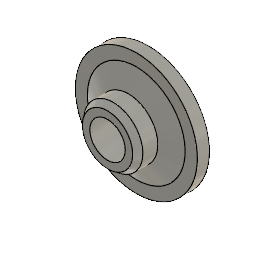
Hexapod (Autodesk Fusion 360 archive; units mm, degrees)
design "Servo Wheel"
Autodesk Fusion 360 part; units mm, degrees
sketch "Profile" plane through (-3.4, -2.5217, -2.4711) normal (-1, 0, 0) x (0, -1, 0)
  line L0 (-59, 21.875) -> (-59, 1.875)
  line L1 (-59, 1.875) -> (-57, 1.875)
  line L2 (-59, 21.875) -> (-57, 21.875)
  line L3 (-57, 21.875) -> (-57, 1.875)
  line L4 (-57, 19.875) -> (-57, 3.875)
  line L5 (-55.7, 16.7) -> (-55.7, 7.05)
  line L6 (-52.2841, 16) -> (-52.3159, 7.75)
  line L7 (-57, 11.875) -> (-55.7, 11.875) construction
  line L8 (-55.7, 11.875) -> (-52.3, 11.875) construction
  line L9 (-57, 19.875) -> (-55.7, 16.7)
  line L10 (-57, 3.875) -> (-55.7, 7.05)
  line L11 (-59, 11.875) -> (-52.3, 11.875)
  line L12 (-55.7, 16.7) -> (-53.2488, 16.7)
  line L13 (-53.2488, 16.7) -> (-52.2841, 16)
  line L14 (-55.7, 7.05) -> (-53.2715, 7.05)
  line L15 (-53.2715, 7.05) -> (-52.3159, 7.75)
  line L16 (-59, 11.875) -> (-52.3, 11.875) construction
  dimension "d77" = 20
  dimension "d78" = 2
  dimension "d79" = 16
  dimension "d80" = 9.65
  dimension "d81" = 8.25
  dimension "d82" = 2
  dimension "d83" = 1.3
  dimension "d84" = 3.4
  dimension "d86" = 0
  dimension "d87" = 0
  dimension "d88" = 0
  dimension "d89" = 0
  dimension "d107" = 0
  dimension "d108" = 0
  dimension "d109" = 0
  dimension "d110" = 0
  dimension "d126" = 0
  dimension "d127" = 0
  dimension "d128" = 0
  dimension "d129" = 0
  dimension "d149" = 0
  dimension "d150" = 0
  dimension "d151" = 0
  dimension "d152" = 0
  dimension "d1" = 6.4
  measures "d77" distance of origin
revolve "Revolve1" add sketch "Profile" angle 360 about axis through (-3.4, 56.4783, 9.4039) along (0, -1, 0) contours L0 L2 L3 L4 L11 | L3 L4 L5 L9 L11 | L5 L6 L11 L12 L13
sketch "Through Hole" plane through (0, 56.4783, 0) normal (0, 1, 0) x (-1, 0, 0)
  circle A0 centre (3.4, 9.4039) radius 10
  circle A1 centre (3.4, 9.4039) radius 2.9
  circle A2 centre (3.4, 9.4039) radius 1.25
  dimension "d98" = 5.8
  dimension "d103" = 2.5
  measures "d98" diameter of A1
  measures "d103" diameter of A2
extrude "Extrude1" cut sketch "Through Hole" against normal through all contours A2
extrude "Extrude2" cut sketch "Through Hole" against normal through all from surface at -2 contours A1

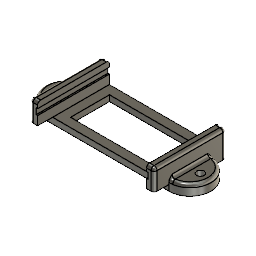
design "Receiver Holder"
Autodesk Fusion 360 part; units mm, degrees
sketch "Profile" plane through (0, 0, 0) normal (0, 1, 0) x (1, 0, 0)
  line L0 (11.5, 0) -> (11.5, -3)
  line L1 (11.5, -3) -> (12, -3)
  line L2 (12, -3) -> (12, -5)
  line L3 (12, -5) -> (11.5, -5)
  line L4 (11.5, -5) -> (11.5, -7)
  line L5 (11.5, -7) -> (14, -7)
  line L6 (14, -7) -> (14, 2)
  line L7 (14, 2) -> (-27.4, 2)
  line L8 (-27.4, 2) -> (-27.4, -7)
  line L9 (-27.4, -7) -> (-24.9, -7)
  line L10 (-24.9, -7) -> (-24.9, -5)
  line L11 (-24.9, -5) -> (-25.4, -5)
  line L12 (-25.4, -5) -> (-25.4, -3)
  line L13 (-25.4, -3) -> (-24.9, -3)
  line L14 (-24.9, -3) -> (-24.9, 0)
  line L15 (-24.9, 0) -> (11.5, 0)
  line L16 (-24.9, 0) -> (-27.4, 0)
  line L17 (11.5, 0) -> (14, 0)
  dimension "d3" = 3
  dimension "d4" = 0.5
  dimension "d5" = 2
  dimension "d6" = 0.5
  dimension "d7" = 2
  dimension "d8" = 2.5
  dimension "d9" = 9
  dimension "d10" = 41.4
  dimension "d11" = 9
  dimension "d12" = 2.5
  dimension "d13" = 2
  dimension "d14" = 0.5
  dimension "d15" = 2
  dimension "d16" = 0.5
  dimension "d33" = 3
extrude "Extrude1" add sketch "Profile" along normal blind 24
sketch "Bottom" plane through (0, 0, -2) normal (0, 0, -1) x (1, 0, 0)
  line L0 (14, 0) -> (-27.4, 0)
  line L1 (-27.4, 0) -> (-27.4, -24)
  line L2 (-27.4, -24) -> (14, -24)
  line L3 (14, -24) -> (14, 0)
  arc A0 (-27.4, -5) -> (-27.4, -19) centre (-27.4, -12) ccw
  arc A1 (14, -19) -> (14, -5) centre (14, -12) ccw
  line L4 (14, -12) -> (17.5, -12) construction
  line L5 (-27.4, -12) -> (-30.9, -12) construction
  circle A2 centre (-30.9, -12) radius 1.25
  circle A3 centre (17.5, -12) radius 1.25
  line L6 (-30.9, -12) -> (17.5, -12) construction
  line L7 (-6.7, -24) -> (-6.7, -21) construction
  line L8 (-27.4, -12) -> (-21.9, -12) construction
  line L9 (-6.7, 0) -> (-6.7, -8) construction
  line L10 (11.5, 0) -> (11.5, -24) construction
  line L11 (14, -12) -> (8.5, -12) construction
  line L12 (-21.9, -21) -> (8.5, -21)
  line L13 (8.5, -21) -> (8.5, -8)
  line L14 (8.5, -8) -> (-21.9, -8)
  line L15 (-21.9, -8) -> (-21.9, -21)
  line L16 (-21.9, -14.5) -> (8.5, -14.5) construction
  line L17 (-6.7, -14.5) -> (-6.7, -12) construction
  dimension "d19" = 7
  dimension "d20" = 7
  dimension "d21" = 3.5
  dimension "d22" = 3.5
  dimension "d23" = 2.5
  dimension "d24" = 2.5
  dimension "d29" = 35
  dimension "d38" = 3
  dimension "d39" = 5.5
  dimension "d40" = 8
  dimension "d41" = 5.5
  dimension "d42" = 13
  dimension "d43" = 30.4
  dimension "d45" = 2.5
  measures "d19" radius of A0
  measures "d20" radius of A1
  measures "d23" diameter of A2
  measures "d24" diameter of A3
  measures "d42" distance of origin
  measures "d43" distance of origin
extrude "Extrude2" add sketch "Bottom" against normal blind 3.5 contours L3 A1 | L1 A0
fillet "Fillet1" radius 1 4 edges at (-27.4, 12, 1.5) (-34.4, 12, 1.5) (14, 12, 1.5) (21, 12, 1.5)
fillet "Fillet2" radius 1 10 edges at (14, 12, 7) (14, 0, 2.5) (-27.4, 12, 7) (-27.4, 0, 2.5) (-26.15, 0, 7) (12.75, 0, 7) (12.75, 24, 7) (14, 24, 2.5) (-27.4, 24, 2.5) (-26.15, 24, 7)
extrude "Extrude3" cut sketch "Bottom" against normal blind 2 contours L12 L13 L14 L15
extrude "Extrude4" cut sketch "Profile" along normal blind 5 contours L6 L7 L8 L15 L16 L17
named bodies: "Receiver Holder"

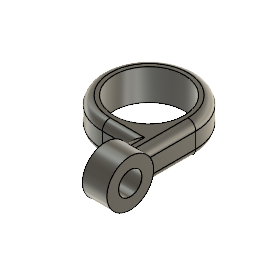
design "Wire Guide"
Autodesk Fusion 360 part; units mm, degrees
sketch "Profile" plane through (0, 0, 0) normal (0, 0, 1) x (1, 0, 0)
  line L0 (2.594, 0) -> (2.594, -6)
  line L1 (2.594, -6) -> (0, -6)
  line L2 (0, -6) -> (0, 0)
  circle A0 centre (-3.406, 6) radius 4.5
  line L3 (2.594, 6) -> (2.594, 0)
  line L4 (0, 0) -> (-3.406, 0)
  arc A1 (2.594, 6) -> (-3.406, 0) centre (-3.406, 6) ccw
  line L5 (2.594, -6) -> (3.175, -6)
  line L6 (3.175, -6) -> (3.175, 0)
  line L7 (3.175, 0) -> (2.594, 0)
  line L8 (2.594, 0) -> (2.594, -6)
  line L9 (3.175, -6) -> (0, -6) construction
  line L10 (0, -6) -> (0, 0) construction
  line L11 (0, 0) -> (3.175, 0) construction
  line L12 (3.175, 0) -> (3.175, -6) construction
  line L13 (2.594, -6) -> (-3.406, -6) construction
  line L14 (-3.406, -6) -> (-3.406, 6) construction
  line L15 (-3.406, 6) -> (2.594, 6) construction
  line L16 (2.594, 6) -> (2.594, -6) construction
  dimension "d38" = 6
  dimension "d39" = 6
  dimension "d40" = 0.581
  dimension "d42" = 6
  dimension "d43" = 3.175
  dimension "d44" = 12
  dimension "d45" = 6
  measures "d38" distance of L2.end
extrude "Extrude1" add sketch "Profile" along normal mid plane 6
sketch "Bottom" plane through (0, 0, 0) normal (1, 0, 0) x (0, 1, 0)
  line L0 (-6, -3) -> (-6, 3) construction
  circle A0 centre (-3, 0) radius 1.5
  circle A1 centre (-3, 0) radius 3
  line L1 (0, -3) -> (12, -3)
  line L2 (12, -3) -> (12, -2)
  line L3 (12, -2) -> (0, -2)
  line L4 (0, -2) -> (0, -3)
  line L5 (0, 3) -> (12, 3)
  line L6 (12, 3) -> (12, 2)
  line L7 (12, 2) -> (0, 2)
  line L8 (0, 2) -> (0, 3)
  line L9 (0, 0) -> (-3, 0) construction
  dimension "d9" = 3
  dimension "d28" = 6
  dimension "d31" = 12
  dimension "d32" = 1
  dimension "d33" = 12
  dimension "d34" = 1
  dimension "d37" = 3
  measures "d9" diameter of A0
  measures "d28" diameter of A1
  measures "d37" distance of L9.start
extrude "Extrude2" cut sketch "Bottom" along normal through all contours A0
extrude "Extrude3" cut sketch "Bottom" along normal through all and the other way through all contours L1 L2 L3 L4 | L5 L6 L7 L8
fillet "Fillet6" radius 3 4 edges at (1.5875, -6, 3) (1.5875, 0, 3) (1.5875, -6, -3) (1.5875, 0, -3)
fillet "Fillet3" radius 1 8 edges at (2.594, 2.618, -2) (-7.6486, 10.2426, -2) (-1.703, 0, -2) (-1.703, 0, 2) (-7.6486, 10.2426, 2) (2.594, 2.618, 2) (0, -0.382, -2) (0, -0.382, 2)
named bodies: "Wire Guide"

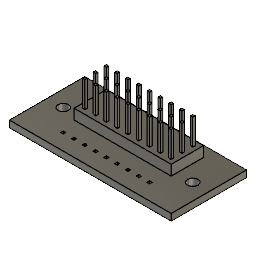
design "Servo Header"
Autodesk Fusion 360 part; units mm, degrees
sketch "Sketch1" plane through (0, 0, 0) normal (0, 0, 1) x (1, 0, 0)
  line L0 (0, 0) -> (2.54, 0)
  line L1 (2.54, 0) -> (2.54, 2.54)
  line L2 (2.54, 2.54) -> (0, 2.54)
  line L3 (0, 2.54) -> (0, 0)
  line L4 (1.57, 0.97) -> (0.97, 0.97)
  line L5 (0.97, 0.97) -> (0.97, 1.57)
  line L6 (0.97, 1.57) -> (1.57, 1.57)
  line L7 (1.57, 1.57) -> (1.57, 0.97)
  line L8 (1.57, 0.97) -> (0.97, 1.57) construction
  line L9 (0.97, 0.97) -> (1.57, 1.57) construction
  line L10 (3.51, 1.57) -> (4.11, 1.57)
  line L11 (3.51, 0.97) -> (4.11, 1.57) construction
  line L12 (4.11, 0.97) -> (3.51, 1.57) construction
  line L13 (4.11, 0.97) -> (3.51, 0.97)
  line L14 (5.08, 0) -> (5.08, 2.54)
  line L15 (3.51, 0.97) -> (3.51, 1.57)
  line L16 (5.08, 2.54) -> (2.54, 2.54)
  line L17 (2.54, 0) -> (5.08, 0)
  line L18 (2.54, 2.54) -> (2.54, 0)
  line L19 (4.11, 1.57) -> (4.11, 0.97)
  line L20 (6.05, 1.57) -> (6.65, 1.57)
  line L21 (6.05, 0.97) -> (6.65, 1.57) construction
  line L22 (6.65, 0.97) -> (6.05, 1.57) construction
  line L23 (6.65, 0.97) -> (6.05, 0.97)
  line L24 (7.62, 0) -> (7.62, 2.54)
  line L25 (6.05, 0.97) -> (6.05, 1.57)
  line L26 (7.62, 2.54) -> (5.08, 2.54)
  line L27 (5.08, 0) -> (7.62, 0)
  line L28 (5.08, 2.54) -> (5.08, 0)
  line L29 (6.65, 1.57) -> (6.65, 0.97)
  line L30 (8.59, 1.57) -> (9.19, 1.57)
  line L31 (8.59, 0.97) -> (9.19, 1.57) construction
  line L32 (9.19, 0.97) -> (8.59, 1.57) construction
  line L33 (9.19, 0.97) -> (8.59, 0.97)
  line L34 (10.16, 0) -> (10.16, 2.54)
  line L35 (8.59, 0.97) -> (8.59, 1.57)
  line L36 (10.16, 2.54) -> (7.62, 2.54)
  line L37 (7.62, 0) -> (10.16, 0)
  line L38 (7.62, 2.54) -> (7.62, 0)
  line L39 (9.19, 1.57) -> (9.19, 0.97)
  line L40 (11.13, 1.57) -> (11.73, 1.57)
  line L41 (11.13, 0.97) -> (11.73, 1.57) construction
  line L42 (11.73, 0.97) -> (11.13, 1.57) construction
  line L43 (11.73, 0.97) -> (11.13, 0.97)
  line L44 (12.7, 0) -> (12.7, 2.54)
  line L45 (11.13, 0.97) -> (11.13, 1.57)
  line L46 (12.7, 2.54) -> (10.16, 2.54)
  line L47 (10.16, 0) -> (12.7, 0)
  line L48 (10.16, 2.54) -> (10.16, 0)
  line L49 (11.73, 1.57) -> (11.73, 0.97)
  line L50 (13.67, 1.57) -> (14.27, 1.57)
  line L51 (13.67, 0.97) -> (14.27, 1.57) construction
  line L52 (14.27, 0.97) -> (13.67, 1.57) construction
  line L53 (14.27, 0.97) -> (13.67, 0.97)
  line L54 (15.24, 0) -> (15.24, 2.54)
  line L55 (13.67, 0.97) -> (13.67, 1.57)
  line L56 (15.24, 2.54) -> (12.7, 2.54)
  line L57 (12.7, 0) -> (15.24, 0)
  line L58 (12.7, 2.54) -> (12.7, 0)
  line L59 (14.27, 1.57) -> (14.27, 0.97)
  line L60 (16.21, 1.57) -> (16.81, 1.57)
  line L61 (16.21, 0.97) -> (16.81, 1.57) construction
  line L62 (16.81, 0.97) -> (16.21, 1.57) construction
  line L63 (16.81, 0.97) -> (16.21, 0.97)
  line L64 (17.78, 0) -> (17.78, 2.54)
  line L65 (16.21, 0.97) -> (16.21, 1.57)
  line L66 (17.78, 2.54) -> (15.24, 2.54)
  line L67 (15.24, 0) -> (17.78, 0)
  line L68 (15.24, 2.54) -> (15.24, 0)
  line L69 (16.81, 1.57) -> (16.81, 0.97)
  line L70 (18.75, 1.57) -> (19.35, 1.57)
  line L71 (18.75, 0.97) -> (19.35, 1.57) construction
  line L72 (19.35, 0.97) -> (18.75, 1.57) construction
  line L73 (19.35, 0.97) -> (18.75, 0.97)
  line L74 (20.32, 0) -> (20.32, 2.54)
  line L75 (18.75, 0.97) -> (18.75, 1.57)
  line L76 (20.32, 2.54) -> (17.78, 2.54)
  line L77 (17.78, 0) -> (20.32, 0)
  line L78 (17.78, 2.54) -> (17.78, 0)
  line L79 (19.35, 1.57) -> (19.35, 0.97)
  line L80 (21.29, 1.57) -> (21.89, 1.57)
  line L81 (21.29, 0.97) -> (21.89, 1.57) construction
  line L82 (21.89, 0.97) -> (21.29, 1.57) construction
  line L83 (21.89, 0.97) -> (21.29, 0.97)
  line L84 (22.86, 0) -> (22.86, 2.54)
  line L85 (21.29, 0.97) -> (21.29, 1.57)
  line L86 (22.86, 2.54) -> (20.32, 2.54)
  line L87 (20.32, 0) -> (22.86, 0)
  line L88 (20.32, 2.54) -> (20.32, 0)
  line L89 (21.89, 1.57) -> (21.89, 0.97)
  line L90 (0.97, 4.11) -> (1.57, 4.11)
  line L91 (0.97, 3.51) -> (1.57, 4.11) construction
  line L92 (1.57, 3.51) -> (0.97, 4.11) construction
  line L93 (1.57, 3.51) -> (0.97, 3.51)
  line L94 (2.54, 2.54) -> (2.54, 5.08)
  line L95 (0.97, 3.51) -> (0.97, 4.11)
  line L96 (2.54, 5.08) -> (0, 5.08)
  line L97 (0, 2.54) -> (2.54, 2.54)
  line L98 (0, 5.08) -> (0, 2.54)
  line L99 (1.57, 4.11) -> (1.57, 3.51)
  line L100 (3.51, 4.11) -> (4.11, 4.11)
  line L101 (3.51, 3.51) -> (4.11, 4.11) construction
  line L102 (4.11, 3.51) -> (3.51, 4.11) construction
  line L103 (4.11, 3.51) -> (3.51, 3.51)
  line L104 (5.08, 2.54) -> (5.08, 5.08)
  line L105 (3.51, 3.51) -> (3.51, 4.11)
  line L106 (5.08, 5.08) -> (2.54, 5.08)
  line L107 (2.54, 2.54) -> (5.08, 2.54)
  line L108 (2.54, 5.08) -> (2.54, 2.54)
  line L109 (4.11, 4.11) -> (4.11, 3.51)
  line L110 (6.05, 4.11) -> (6.65, 4.11)
  line L111 (6.05, 3.51) -> (6.65, 4.11) construction
  line L112 (6.65, 3.51) -> (6.05, 4.11) construction
  line L113 (6.65, 3.51) -> (6.05, 3.51)
  line L114 (7.62, 2.54) -> (7.62, 5.08)
  line L115 (6.05, 3.51) -> (6.05, 4.11)
  line L116 (7.62, 5.08) -> (5.08, 5.08)
  line L117 (5.08, 2.54) -> (7.62, 2.54)
  line L118 (5.08, 5.08) -> (5.08, 2.54)
  line L119 (6.65, 4.11) -> (6.65, 3.51)
  line L120 (8.59, 4.11) -> (9.19, 4.11)
  line L121 (8.59, 3.51) -> (9.19, 4.11) construction
  line L122 (9.19, 3.51) -> (8.59, 4.11) construction
  line L123 (9.19, 3.51) -> (8.59, 3.51)
  line L124 (10.16, 2.54) -> (10.16, 5.08)
  line L125 (8.59, 3.51) -> (8.59, 4.11)
  line L126 (10.16, 5.08) -> (7.62, 5.08)
  line L127 (7.62, 2.54) -> (10.16, 2.54)
  line L128 (7.62, 5.08) -> (7.62, 2.54)
  line L129 (9.19, 4.11) -> (9.19, 3.51)
  line L130 (11.13, 4.11) -> (11.73, 4.11)
  line L131 (11.13, 3.51) -> (11.73, 4.11) construction
  line L132 (11.73, 3.51) -> (11.13, 4.11) construction
  line L133 (11.73, 3.51) -> (11.13, 3.51)
  line L134 (12.7, 2.54) -> (12.7, 5.08)
  line L135 (11.13, 3.51) -> (11.13, 4.11)
  line L136 (12.7, 5.08) -> (10.16, 5.08)
  line L137 (10.16, 2.54) -> (12.7, 2.54)
  line L138 (10.16, 5.08) -> (10.16, 2.54)
  line L139 (11.73, 4.11) -> (11.73, 3.51)
  line L140 (13.67, 4.11) -> (14.27, 4.11)
  line L141 (13.67, 3.51) -> (14.27, 4.11) construction
  line L142 (14.27, 3.51) -> (13.67, 4.11) construction
  line L143 (14.27, 3.51) -> (13.67, 3.51)
  line L144 (15.24, 2.54) -> (15.24, 5.08)
  line L145 (13.67, 3.51) -> (13.67, 4.11)
  line L146 (15.24, 5.08) -> (12.7, 5.08)
  line L147 (12.7, 2.54) -> (15.24, 2.54)
  line L148 (12.7, 5.08) -> (12.7, 2.54)
  line L149 (14.27, 4.11) -> (14.27, 3.51)
  line L150 (16.21, 4.11) -> (16.81, 4.11)
  line L151 (16.21, 3.51) -> (16.81, 4.11) construction
  line L152 (16.81, 3.51) -> (16.21, 4.11) construction
  line L153 (16.81, 3.51) -> (16.21, 3.51)
  line L154 (17.78, 2.54) -> (17.78, 5.08)
  line L155 (16.21, 3.51) -> (16.21, 4.11)
  line L156 (17.78, 5.08) -> (15.24, 5.08)
  line L157 (15.24, 2.54) -> (17.78, 2.54)
  line L158 (15.24, 5.08) -> (15.24, 2.54)
  line L159 (16.81, 4.11) -> (16.81, 3.51)
  line L160 (18.75, 4.11) -> (19.35, 4.11)
  line L161 (18.75, 3.51) -> (19.35, 4.11) construction
  line L162 (19.35, 3.51) -> (18.75, 4.11) construction
  line L163 (19.35, 3.51) -> (18.75, 3.51)
  line L164 (20.32, 2.54) -> (20.32, 5.08)
  line L165 (18.75, 3.51) -> (18.75, 4.11)
  line L166 (20.32, 5.08) -> (17.78, 5.08)
  line L167 (17.78, 2.54) -> (20.32, 2.54)
  line L168 (17.78, 5.08) -> (17.78, 2.54)
  line L169 (19.35, 4.11) -> (19.35, 3.51)
  line L170 (21.29, 4.11) -> (21.89, 4.11)
  line L171 (21.29, 3.51) -> (21.89, 4.11) construction
  line L172 (21.89, 3.51) -> (21.29, 4.11) construction
  line L173 (21.89, 3.51) -> (21.29, 3.51)
  line L174 (22.86, 2.54) -> (22.86, 5.08)
  line L175 (21.29, 3.51) -> (21.29, 4.11)
  line L176 (22.86, 5.08) -> (20.32, 5.08)
  line L177 (20.32, 2.54) -> (22.86, 2.54)
  line L178 (20.32, 5.08) -> (20.32, 2.54)
  line L179 (21.89, 4.11) -> (21.89, 3.51)
  line L180 (0.97, 6.65) -> (1.57, 6.65)
  line L181 (0.97, 6.05) -> (1.57, 6.65) construction
  line L182 (1.57, 6.05) -> (0.97, 6.65) construction
  line L183 (1.57, 6.05) -> (0.97, 6.05)
  line L184 (2.54, 5.08) -> (2.54, 7.62)
  line L185 (0.97, 6.05) -> (0.97, 6.65)
  line L186 (2.54, 7.62) -> (0, 7.62)
  line L187 (0, 5.08) -> (2.54, 5.08)
  line L188 (0, 7.62) -> (0, 5.08)
  line L189 (1.57, 6.65) -> (1.57, 6.05)
  line L190 (3.51, 6.65) -> (4.11, 6.65)
  line L191 (3.51, 6.05) -> (4.11, 6.65) construction
  line L192 (4.11, 6.05) -> (3.51, 6.65) construction
  line L193 (4.11, 6.05) -> (3.51, 6.05)
  line L194 (5.08, 5.08) -> (5.08, 7.62)
  line L195 (3.51, 6.05) -> (3.51, 6.65)
  line L196 (5.08, 7.62) -> (2.54, 7.62)
  line L197 (2.54, 5.08) -> (5.08, 5.08)
  line L198 (2.54, 7.62) -> (2.54, 5.08)
  line L199 (4.11, 6.65) -> (4.11, 6.05)
  line L200 (6.05, 6.65) -> (6.65, 6.65)
  line L201 (6.05, 6.05) -> (6.65, 6.65) construction
  line L202 (6.65, 6.05) -> (6.05, 6.65) construction
  line L203 (6.65, 6.05) -> (6.05, 6.05)
  line L204 (7.62, 5.08) -> (7.62, 7.62)
  line L205 (6.05, 6.05) -> (6.05, 6.65)
  line L206 (7.62, 7.62) -> (5.08, 7.62)
  line L207 (5.08, 5.08) -> (7.62, 5.08)
  line L208 (5.08, 7.62) -> (5.08, 5.08)
  line L209 (6.65, 6.65) -> (6.65, 6.05)
  line L210 (8.59, 6.65) -> (9.19, 6.65)
  line L211 (8.59, 6.05) -> (9.19, 6.65) construction
  line L212 (9.19, 6.05) -> (8.59, 6.65) construction
  line L213 (9.19, 6.05) -> (8.59, 6.05)
  line L214 (10.16, 5.08) -> (10.16, 7.62)
  line L215 (8.59, 6.05) -> (8.59, 6.65)
  line L216 (10.16, 7.62) -> (7.62, 7.62)
  line L217 (7.62, 5.08) -> (10.16, 5.08)
  line L218 (7.62, 7.62) -> (7.62, 5.08)
  line L219 (9.19, 6.65) -> (9.19, 6.05)
  line L220 (11.13, 6.65) -> (11.73, 6.65)
  line L221 (11.13, 6.05) -> (11.73, 6.65) construction
  line L222 (11.73, 6.05) -> (11.13, 6.65) construction
  line L223 (11.73, 6.05) -> (11.13, 6.05)
  line L224 (12.7, 5.08) -> (12.7, 7.62)
  line L225 (11.13, 6.05) -> (11.13, 6.65)
  line L226 (12.7, 7.62) -> (10.16, 7.62)
  line L227 (10.16, 5.08) -> (12.7, 5.08)
  line L228 (10.16, 7.62) -> (10.16, 5.08)
  line L229 (11.73, 6.65) -> (11.73, 6.05)
  line L230 (13.67, 6.65) -> (14.27, 6.65)
  line L231 (13.67, 6.05) -> (14.27, 6.65) construction
  line L232 (14.27, 6.05) -> (13.67, 6.65) construction
  line L233 (14.27, 6.05) -> (13.67, 6.05)
  line L234 (15.24, 5.08) -> (15.24, 7.62)
  line L235 (13.67, 6.05) -> (13.67, 6.65)
  line L236 (15.24, 7.62) -> (12.7, 7.62)
  line L237 (12.7, 5.08) -> (15.24, 5.08)
  line L238 (12.7, 7.62) -> (12.7, 5.08)
  line L239 (14.27, 6.65) -> (14.27, 6.05)
  line L240 (16.21, 6.65) -> (16.81, 6.65)
  line L241 (16.21, 6.05) -> (16.81, 6.65) construction
  line L242 (16.81, 6.05) -> (16.21, 6.65) construction
  line L243 (16.81, 6.05) -> (16.21, 6.05)
  line L244 (17.78, 5.08) -> (17.78, 7.62)
  line L245 (16.21, 6.05) -> (16.21, 6.65)
  line L246 (17.78, 7.62) -> (15.24, 7.62)
  line L247 (15.24, 5.08) -> (17.78, 5.08)
  line L248 (15.24, 7.62) -> (15.24, 5.08)
  line L249 (16.81, 6.65) -> (16.81, 6.05)
  line L250 (18.75, 6.65) -> (19.35, 6.65)
  line L251 (18.75, 6.05) -> (19.35, 6.65) construction
  line L252 (19.35, 6.05) -> (18.75, 6.65) construction
  line L253 (19.35, 6.05) -> (18.75, 6.05)
  line L254 (20.32, 5.08) -> (20.32, 7.62)
  line L255 (18.75, 6.05) -> (18.75, 6.65)
  line L256 (20.32, 7.62) -> (17.78, 7.62)
  line L257 (17.78, 5.08) -> (20.32, 5.08)
  line L258 (17.78, 7.62) -> (17.78, 5.08)
  line L259 (19.35, 6.65) -> (19.35, 6.05)
  line L260 (21.29, 6.65) -> (21.89, 6.65)
  line L261 (21.29, 6.05) -> (21.89, 6.65) construction
  line L262 (21.89, 6.05) -> (21.29, 6.65) construction
  line L263 (21.89, 6.05) -> (21.29, 6.05)
  line L264 (22.86, 5.08) -> (22.86, 7.62)
  line L265 (21.29, 6.05) -> (21.29, 6.65)
  line L266 (22.86, 7.62) -> (20.32, 7.62)
  line L267 (20.32, 5.08) -> (22.86, 5.08)
  line L268 (20.32, 7.62) -> (20.32, 5.08)
  line L269 (21.89, 6.65) -> (21.89, 6.05)
  line L270 (0, 0) -> (0, -7.62) construction
  line L271 (0, 7.62) -> (0, 10.16) construction
  line L272 (22.86, 0) -> (30.48, 0) construction
  line L273 (0, 0) -> (-7.62, 0) construction
  line L274 (-7.62, -7.62) -> (30.48, -7.62)
  line L275 (30.48, -7.62) -> (30.48, 10.16)
  line L276 (30.48, 10.16) -> (-7.62, 10.16)
  line L277 (-7.62, 10.16) -> (-7.62, -7.62)
  circle A0 centre (26.67, 1.27) radius 1.2
  circle A1 centre (-3.81, 1.27) radius 1.2
  line L278 (-7.62, 1.27) -> (-3.81, 1.27) construction
  line L279 (30.48, 1.27) -> (26.67, 1.27) construction
  line L280 (1.57, -4.11) -> (0.97, -3.51) construction
  line L281 (1.57, -3.51) -> (1.57, -4.11)
  line L282 (1.57, -4.11) -> (0.97, -4.11)
  line L283 (0.97, -4.11) -> (1.57, -3.51) construction
  line L284 (0.97, -4.11) -> (0.97, -3.51)
  line L285 (0.97, -3.51) -> (1.57, -3.51)
  line L286 (4.11, -4.11) -> (3.51, -4.11)
  line L287 (3.51, -3.51) -> (4.11, -3.51)
  line L288 (4.11, -4.11) -> (3.51, -3.51) construction
  line L289 (3.51, -4.11) -> (3.51, -3.51)
  line L290 (3.51, -4.11) -> (4.11, -3.51) construction
  line L291 (4.11, -3.51) -> (4.11, -4.11)
  line L292 (6.05, -3.51) -> (6.65, -3.51)
  line L293 (6.05, -4.11) -> (6.05, -3.51)
  line L294 (6.65, -4.11) -> (6.05, -3.51) construction
  line L295 (6.65, -3.51) -> (6.65, -4.11)
  line L296 (6.65, -4.11) -> (6.05, -4.11)
  line L297 (6.05, -4.11) -> (6.65, -3.51) construction
  line L298 (8.59, -4.11) -> (8.59, -3.51)
  line L299 (9.19, -3.51) -> (9.19, -4.11)
  line L300 (9.19, -4.11) -> (8.59, -3.51) construction
  line L301 (8.59, -4.11) -> (9.19, -3.51) construction
  line L302 (8.59, -3.51) -> (9.19, -3.51)
  line L303 (9.19, -4.11) -> (8.59, -4.11)
  line L304 (11.13, -4.11) -> (11.73, -3.51) construction
  line L305 (11.73, -3.51) -> (11.73, -4.11)
  line L306 (11.73, -4.11) -> (11.13, -3.51) construction
  line L307 (11.73, -4.11) -> (11.13, -4.11)
  line L308 (11.13, -4.11) -> (11.13, -3.51)
  line L309 (11.13, -3.51) -> (11.73, -3.51)
  line L310 (14.27, -4.11) -> (13.67, -4.11)
  line L311 (13.67, -4.11) -> (14.27, -3.51) construction
  line L312 (14.27, -4.11) -> (13.67, -3.51) construction
  line L313 (13.67, -3.51) -> (14.27, -3.51)
  line L314 (13.67, -4.11) -> (13.67, -3.51)
  line L315 (14.27, -3.51) -> (14.27, -4.11)
  line L316 (16.21, -4.11) -> (16.21, -3.51)
  line L317 (16.81, -3.51) -> (16.81, -4.11)
  line L318 (16.21, -4.11) -> (16.81, -3.51) construction
  line L319 (16.81, -4.11) -> (16.21, -4.11)
  line L320 (16.21, -3.51) -> (16.81, -3.51)
  line L321 (16.81, -4.11) -> (16.21, -3.51) construction
  line L322 (18.75, -4.11) -> (19.35, -3.51) construction
  line L323 (18.75, -3.51) -> (19.35, -3.51)
  line L324 (19.35, -3.51) -> (19.35, -4.11)
  line L325 (19.35, -4.11) -> (18.75, -3.51) construction
  line L326 (18.75, -4.11) -> (18.75, -3.51)
  line L327 (19.35, -4.11) -> (18.75, -4.11)
  line L328 (21.89, -4.11) -> (21.29, -4.11)
  line L329 (21.29, -4.11) -> (21.29, -3.51)
  line L330 (21.89, -3.51) -> (21.89, -4.11)
  line L331 (21.29, -3.51) -> (21.89, -3.51)
  line L332 (21.89, -4.11) -> (21.29, -3.51) construction
  line L333 (21.29, -4.11) -> (21.89, -3.51) construction
  point P0 (-350.72, -350.72)
  point P1 (0, -350.72)
  dimension "d9" = 7.62
  dimension "d10" = 2.54
  dimension "d12" = 7.62
  dimension "d13" = 7.62
  dimension "d16" = 2.4
  dimension "d17" = 2.4
  dimension "d24" = 3.81
  dimension "d25" = 3.81
  dimension "d28" = 0
  dimension "d29" = -5.08
  measures "d9" distance of L0.start
  measures "d13" distance of L0.start
  measures "d16" diameter of A0
  measures "d17" diameter of A1
extrude "Extrude1" add sketch "Sketch1" along normal blind 1.6 contours L274 L275 L276 L277 | L281 L282 L284 L285 | L286 L287 L289 L291 | L292 L293 L295 L296 | L298 L299 L302 L303 | L305 L307 L308 L309 | L310 L313 L314 L315 | L316 L317 L319 L320 | L323 L324 L326 L327 | L328 L329 L330 L331
extrude "Extrude2" add sketch "Sketch1" along normal blind 4 contours L0 L1 L2 L3 L18 L97 | L1 L14 L16 L17 L18 L28 L107 | L2 L94 L96 L97 L98 L108 L187 | L16 L94 L104 L106 L107 L108 L118 L197 | L14 L24 L26 L27 L28 L38 L117 | L96 L184 L186 L187 L188 L198 | L26 L104 L114 L116 L117 L118 L128 L207 | L106 L184 L194 L196 L197 L198 L208 | L24 L34 L36 L37 L38 L48 L127 | L36 L114 L124 L126 L127 L128 L138 L217 | L116 L194 L204 L206 L207 L208 L218 | L34 L44 L46 L47 L48 L58 L137 | L46 L124 L134 L136 L137 L138 L148 L227 | L126 L204 L214 L216 L217 L218 L228 | L44 L54 L56 L57 L58 L68 L147 | L56 L134 L144 L146 L147 L148 L158 L237 | L136 L214 L224 L226 L227 L228 L238 | L54 L64 L66 L67 L68 L78 L157 | L66 L144 L154 L156 L157 L158 L168 L247 | L146 L224 L234 L236 L237 L238 L248 | L64 L74 L76 L77 L78 L88 L167 | L76 L154 L164 L166 L167 L168 L178 L257 | L156 L234 L244 L246 L247 L248 L258 | L74 L84 L86 L87 L88 L177 | L86 L164 L174 L176 L177 L178 L267 | L166 L244 L254 L256 L257 L258 L268 | L176 L254 L264 L266 L267 L268
extrude "Extrude3" add sketch "Sketch1" along normal blind 10.1 contours L4 L5 L6 L7 | L10 L13 L15 L19 | L20 L23 L25 L29 | L30 L33 L35 L39 | L40 L43 L45 L49 | L50 L53 L55 L59 | L60 L63 L65 L69 | L70 L73 L75 L79 | L80 L83 L85 L89 | L90 L93 L95 L99 | L100 L103 L105 L109 | L110 L113 L115 L119 | L120 L123 L125 L129 | L130 L133 L135 L139 | L140 L143 L145 L149 | L150 L153 L155 L159 | L160 L163 L165 L169 | L170 L173 L175 L179 | L180 L183 L185 L189 | L190 L193 L195 L199 | L200 L203 L205 L209 | L210 L213 L215 L219 | L220 L223 L225 L229 | L230 L233 L235 L239 | L240 L243 L245 L249 | L250 L253 L255 L259 | L260 L263 L265 L269
extrude "Extrude4" cut sketch "Sketch1" along normal through all contours L281 L282 L284 L285 | L286 L287 L289 L291 | L292 L293 L295 L296 | L298 L299 L302 L303 | L305 L307 L308 L309 | L310 L313 L314 L315 | L316 L317 L319 L320 | L323 L324 L326 L327 | L328 L329 L330 L331
equation "d9 = 2.54 mm * 3"
equation "d12 = ( 2.54 * 3 ) * 1 mm"
equation "d13 = ( 2.54 * 3 ) * 1 mm"
equation "d20 = 1.6 mm + 2.4 mm"
equation "d22 = 1.6 mm + 8.5 mm"
equation "d24 = ( 2.54 * 1.5 ) * 1 mm"
equation "d25 = ( 2.54 * 1.5 ) * 1 mm"
equation "d29 = ( -2.54 * 2 ) * 1 mm"

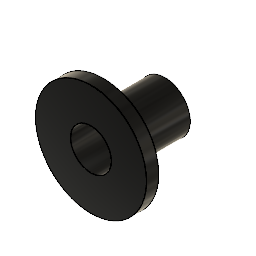
design "Bearing Center"
Autodesk Fusion 360 part; units mm, degrees
sketch "Sketch1" plane through (0, 0, 0) normal (0, 1, 0) x (1, 0, 0)
  circle A0 centre (0, 0) radius 2.05
  circle A1 centre (0, 0) radius 1.65
  circle A2 centre (0, 0) radius 4.5
  dimension "d1" = 4.1
  dimension "d2" = 3.3
  dimension "d3" = 9
  measures "d1" diameter of A0
  measures "d2" diameter of A1
  measures "d3" diameter of A2
extrude "Extrude1" add sketch "Sketch1" along normal blind 6 contours A0
extrude "Extrude2" add sketch "Sketch1" along normal blind 1 contours A2
named bodies: "Bearing Center"

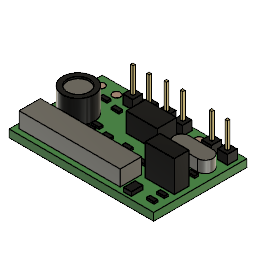
design "Receiver"
Autodesk Fusion 360 part; units mm, degrees
sketch "Sketch1" plane through (0, 0, 0) normal (0, 0, 1) x (1, 0, 0)
  line L0 (18.6, -12) -> (-18.6, -12)
  line L1 (-18.6, -12) -> (-18.6, 12)
  line L2 (-18.6, 12) -> (18.6, 12)
  line L3 (18.6, 12) -> (18.6, -12)
  line L4 (-18.6, -12) -> (-17.3635, -12) construction
  line L5 (-18.6, -10.65) -> (-18.6, -12) construction
  line L6 (-17.3635, -10.65) -> (8.6365, -10.65)
  line L7 (8.6365, -10.65) -> (8.6365, -5.15)
  line L8 (8.6365, -5.15) -> (-17.3635, -5.15)
  line L9 (-17.3635, -5.15) -> (-17.3635, -10.65)
  circle A0 centre (-13.3452, 0.5737) radius 4.075
  circle A1 centre (-13.3452, 0.5737) radius 2.8242
  line L10 (9.7824, -1.5868) -> (17.2824, -1.5868)
  line L11 (17.2824, -1.5868) -> (17.2824, -5.3868)
  line L12 (17.2824, -5.3868) -> (9.7824, -5.3868)
  line L13 (9.7824, -5.3868) -> (9.7824, -1.5868)
  line L14 (10.1467, -8.3154) -> (12.1467, -8.3154)
  line L15 (12.1467, -8.3154) -> (12.1467, -11.3154)
  line L16 (12.1467, -11.3154) -> (10.1467, -11.3154)
  line L17 (10.1467, -11.3154) -> (10.1467, -8.3154)
  line L18 (-7.0489, -3.1736) -> (-2.0489, -3.1736)
  line L19 (-2.0489, -3.1736) -> (-2.0489, -5.1736)
  line L20 (-2.0489, -5.1736) -> (-7.0489, -5.1736)
  line L21 (-7.0489, -5.1736) -> (-7.0489, -3.1736)
  line L22 (9.1707, 6.6458) -> (15.17, 6.6458)
  line L23 (17.17, 4.6511) -> (17.17, 4.6511)
  line L24 (15.17, 2.6458) -> (9.1707, 2.6458)
  line L25 (7.1707, 4.6401) -> (7.1707, 4.6401)
  arc A2 (9.1707, 6.6458) -> (7.1707, 4.6401) centre (9.1707, 4.6458) ccw
  arc A3 (7.1707, 4.6401) -> (9.1707, 2.6458) centre (9.1707, 4.6458) ccw
  arc A4 (17.17, 4.6511) -> (15.17, 6.6458) centre (15.17, 4.6458) ccw
  arc A5 (15.17, 2.6458) -> (17.17, 4.6511) centre (15.17, 4.6458) ccw
  line L26 (15.029, 7.9882) -> (17.569, 7.9882)
  line L27 (17.569, 7.9882) -> (17.569, 10.5282)
  line L28 (17.569, 10.5282) -> (15.029, 10.5282)
  line L29 (15.029, 10.5282) -> (15.029, 7.9882)
  line L30 (-5.2876, 10.5822) -> (-2.7476, 10.5822)
  line L31 (-2.7476, 10.5822) -> (-2.7476, 8.0422)
  line L32 (-2.7476, 8.0422) -> (-5.2876, 8.0422)
  line L33 (-5.2876, 8.0422) -> (-5.2876, 10.5822)
  line L34 (-9.3461, 10.5822) -> (-6.8061, 10.5822)
  line L35 (-6.8061, 10.5822) -> (-6.8061, 8.0422)
  line L36 (-6.8061, 8.0422) -> (-9.3461, 8.0422)
  line L37 (-9.3461, 8.0422) -> (-9.3461, 10.5822)
  line L38 (2.7807, 11.1689) -> (5.3207, 11.1689)
  line L39 (5.3207, 11.1689) -> (5.3207, 8.6289)
  line L40 (5.3207, 8.6289) -> (2.7807, 8.6289)
  line L41 (2.7807, 8.6289) -> (2.7807, 11.1689)
  line L42 (-1.3638, 11.2107) -> (1.1762, 11.2107)
  line L43 (1.1762, 11.2107) -> (1.1762, 8.6707)
  line L44 (1.1762, 8.6707) -> (-1.3638, 8.6707)
  line L45 (-1.3638, 8.6707) -> (-1.3638, 11.2107)
  line L46 (10.9956, 10.4785) -> (13.5356, 10.4785)
  line L47 (13.5356, 10.4785) -> (13.5356, 7.9385)
  line L48 (13.5356, 7.9385) -> (10.9956, 7.9385)
  line L49 (10.9956, 7.9385) -> (10.9956, 10.4785)
  line L50 (-2.5723, 7.0984) -> (5.4277, 7.0984)
  line L51 (5.4277, 7.0984) -> (5.4277, 2.0984)
  line L52 (5.4277, 2.0984) -> (-2.5723, 2.0984)
  line L53 (-2.5723, 2.0984) -> (-2.5723, 7.0984)
  circle A6 centre (-12.317, 9.3785) radius 1
  circle A7 centre (-16.3775, 9.3902) radius 1
  circle A8 centre (8.3691, 9.8873) radius 1
  line L54 (-13.7071, 7.3102) -> (-11.7071, 7.3102)
  line L55 (-11.7071, 7.3102) -> (-11.7071, 6.3102)
  line L56 (-11.7071, 6.3102) -> (-13.7071, 6.3102)
  line L57 (-13.7071, 6.3102) -> (-13.7071, 7.3102)
  line L58 (-9.7657, 6.4316) -> (-7.7657, 6.4316)
  line L59 (-7.7657, 6.4316) -> (-7.7657, 5.4316)
  line L60 (-7.7657, 5.4316) -> (-9.7657, 5.4316)
  line L61 (-9.7657, 5.4316) -> (-9.7657, 6.4316)
  line L62 (-8.8702, 0.4569) -> (-6.8702, 0.4569)
  line L63 (-6.8702, 0.4569) -> (-6.8702, -0.5431)
  line L64 (-6.8702, -0.5431) -> (-8.8702, -0.5431)
  line L65 (-8.8702, -0.5431) -> (-8.8702, 0.4569)
  line L66 (-9.1462, -1.1246) -> (-7.1462, -1.1246)
  line L67 (-7.1462, -1.1246) -> (-7.1462, -2.1246)
  line L68 (-7.1462, -2.1246) -> (-9.1462, -2.1246)
  line L69 (-9.1462, -2.1246) -> (-9.1462, -1.1246)
  line L70 (-10.0397, -2.7377) -> (-8.0397, -2.7377)
  line L71 (-8.0397, -2.7377) -> (-8.0397, -3.7377)
  line L72 (-8.0397, -3.7377) -> (-10.0397, -3.7377)
  line L73 (-10.0397, -3.7377) -> (-10.0397, -2.7377)
  line L74 (-5.0122, -0.656) -> (-3.0122, -0.656)
  line L75 (-3.0122, -0.656) -> (-3.0122, -1.656)
  line L76 (-3.0122, -1.656) -> (-5.0122, -1.656)
  line L77 (-5.0122, -1.656) -> (-5.0122, -0.656)
  line L78 (0.0422, -3.3505) -> (2.0422, -3.3505)
  line L79 (2.0422, -3.3505) -> (2.0422, -4.3505)
  line L80 (2.0422, -4.3505) -> (0.0422, -4.3505)
  line L81 (0.0422, -4.3505) -> (0.0422, -3.3505)
  line L82 (-0.0539, -0.5974) -> (1.9461, -0.5974)
  line L83 (1.9461, -0.5974) -> (1.9461, -1.5974)
  line L84 (1.9461, -1.5974) -> (-0.0539, -1.5974)
  line L85 (-0.0539, -1.5974) -> (-0.0539, -0.5974)
  line L86 (5.1762, -4.1119) -> (7.1762, -4.1119)
  line L87 (7.1762, -4.1119) -> (7.1762, -5.1119)
  line L88 (7.1762, -5.1119) -> (5.1762, -5.1119)
  line L89 (5.1762, -5.1119) -> (5.1762, -4.1119)
  line L90 (5.0934, -1.917) -> (7.0934, -1.917)
  line L91 (7.0934, -1.917) -> (7.0934, -2.917)
  line L92 (7.0934, -2.917) -> (5.0934, -2.917)
  line L93 (5.0934, -2.917) -> (5.0934, -1.917)
  line L94 (8.3737, 7.9822) -> (10.3737, 7.9822)
  line L95 (10.3737, 7.9822) -> (10.3737, 6.9822)
  line L96 (10.3737, 6.9822) -> (8.3737, 6.9822)
  line L97 (8.3737, 6.9822) -> (8.3737, 7.9822)
  line L98 (14.8169, -9.126) -> (16.8169, -9.126)
  line L99 (16.8169, -9.126) -> (16.8169, -10.126)
  line L100 (16.8169, -10.126) -> (14.8169, -10.126)
  line L101 (14.8169, -10.126) -> (14.8169, -9.126)
  line L102 (14.8755, -6.5445) -> (16.8755, -6.5445)
  line L103 (16.8755, -6.5445) -> (16.8755, -7.5445)
  line L104 (16.8755, -7.5445) -> (14.8755, -7.5445)
  line L105 (14.8755, -7.5445) -> (14.8755, -6.5445)
  line L106 (14.2898, 1.8318) -> (16.2898, 1.8318)
  line L107 (16.2898, 1.8318) -> (16.2898, 0.8318)
  line L108 (16.2898, 0.8318) -> (14.2898, 0.8318)
  line L109 (14.2898, 0.8318) -> (14.2898, 1.8318)
  line L110 (5.7378, 2.2418) -> (6.7378, 2.2418)
  line L111 (6.7378, 2.2418) -> (6.7378, 0.2418)
  line L112 (6.7378, 0.2418) -> (5.7378, 0.2418)
  line L113 (5.7378, 0.2418) -> (5.7378, 2.2418)
  line L114 (5.8549, 5.3463) -> (6.8549, 5.3463)
  line L115 (6.8549, 5.3463) -> (6.8549, 3.3463)
  line L116 (6.8549, 3.3463) -> (5.8549, 3.3463)
  line L117 (5.8549, 3.3463) -> (5.8549, 5.3463)
  line L118 (5.9135, 7.8651) -> (6.9135, 7.8651)
  line L119 (6.9135, 7.8651) -> (6.9135, 5.8651)
  line L120 (6.9135, 5.8651) -> (5.9135, 5.8651)
  line L121 (5.9135, 5.8651) -> (5.9135, 7.8651)
  line L122 (-17.3635, -3.4986) -> (-15.3635, -3.4986)
  line L123 (-15.3635, -3.4986) -> (-15.3635, -4.4986)
  line L124 (-15.3635, -4.4986) -> (-17.3635, -4.4986)
  line L125 (-17.3635, -4.4986) -> (-17.3635, -3.4986)
  line L126 (-8.353, 9.6467) -> (-7.703, 9.6467)
  line L127 (-7.703, 9.6467) -> (-7.703, 8.9967)
  line L128 (-7.703, 8.9967) -> (-8.353, 8.9967)
  line L129 (-8.353, 8.9967) -> (-8.353, 9.6467)
  line L130 (-3.6201, 9.0505) -> (-4.2701, 9.0505)
  line L131 (-4.2701, 9.0505) -> (-4.2701, 9.7005)
  line L132 (-3.6201, 9.7005) -> (-3.6201, 9.0505)
  line L133 (-4.2701, 9.7005) -> (-3.6201, 9.7005)
  line L134 (0.2479, 9.6414) -> (-0.4021, 9.6414)
  line L135 (0.2479, 10.2914) -> (0.2479, 9.6414)
  line L136 (3.7882, 10.2914) -> (4.4382, 10.2914)
  line L137 (4.4382, 9.6414) -> (3.7882, 9.6414)
  line L138 (4.4382, 10.2914) -> (4.4382, 9.6414)
  line L139 (-0.4021, 9.6414) -> (-0.4021, 10.2914)
  line L140 (3.7882, 9.6414) -> (3.7882, 10.2914)
  line L141 (-0.4021, 10.2914) -> (0.2479, 10.2914)
  line L142 (11.9539, 9.593) -> (12.6039, 9.593)
  line L143 (12.6039, 8.943) -> (11.9539, 8.943)
  line L144 (16.0367, 8.8893) -> (16.0367, 9.5393)
  line L145 (11.9539, 8.943) -> (11.9539, 9.593)
  line L146 (16.6867, 8.8893) -> (16.0367, 8.8893)
  line L147 (16.0367, 9.5393) -> (16.6867, 9.5393)
  line L148 (16.6867, 9.5393) -> (16.6867, 8.8893)
  line L149 (12.6039, 9.593) -> (12.6039, 8.943)
extrude "Extrude1" add sketch "Sketch1" along normal blind 2 contours L0 L1 L2 L3 makes body 1
extrude "Extrude2" add sketch "Sketch1" along normal blind 2.5 separate body contours L54 L55 L56 L57 | L58 L59 L60 L61 | L62 L63 L64 L65 | L66 L67 L68 L69 | L70 L71 L72 L73 | L74 L75 L76 L77 | L78 L79 L80 L81 | L82 L83 L84 L85 | L86 L87 L88 L89 | L90 L91 L92 L93 | L94 L95 L96 L97 | L98 L99 L100 L101 | L102 L103 L104 L105 | L106 L107 L108 L109 | L110 L111 L112 L113 | L114 L115 L116 L117 | L118 L119 L120 L121 | L122 L123 L124 L125 makes body 2 at (-16.6968, -3.4986, 0.8333) makes body 3 at (-4.3455, -0.656, 0.8333) makes body 4 at (5.7601, -1.917, 0.8333) makes body 5 at (6.8549, 4.6797, 0.8333) makes body 6 at (-13.0405, 7.3102, 0.8333) makes body 7 at (6.7378, 1.5752, 0.8333) makes body 8 at (5.8429, -4.1119, 0.8333) makes body 9 at (-8.2035, 0.4569, 0.8333) makes body 10 at (15.5422, -6.5445, 0.8333) makes body 11 at (-9.373, -2.7377, 0.8333) makes body 12 at (0.6128, -0.5974, 0.8333) makes body 13 at (14.9564, 1.8318, 0.8333) makes body 14 at (6.9135, 7.1984, 0.8333) makes body 15 at (-9.099, 6.4316, 0.8333) makes body 16 at (9.0403, 7.9822, 0.8333) makes body 17 at (0.7089, -3.3505, 0.8333) makes body 18 at (-8.4795, -1.1246, 0.8333) makes body 19 at (15.4836, -9.126, 0.8333)
extrude "Extrude3" add sketch "Sketch1" along normal blind 11 separate body contours L126 L127 L128 L129 | L130 L131 L132 L133 | L134 L135 L139 L141 | L136 L137 L138 L140 | L142 L143 L145 L149 | L144 L146 L147 L148 makes body 20 at (4.4382, 10.0747, 3.6667) makes body 21 at (-8.353, 9.2134, 3.6667) makes body 22 at (12.1705, 9.593, 3.6667) makes body 23 at (0.2479, 10.0747, 3.6667) makes body 24 at (-3.6201, 9.4838, 3.6667) makes body 25 at (16.0367, 9.106, 3.6667)
extrude "Extrude4" add sketch "Sketch1" along normal blind 4.4 separate body contours L26 L27 L28 L29 | L30 L31 L32 L33 | L34 L35 L36 L37 | L38 L39 L40 L41 | L42 L43 L44 L45 | L46 L47 L48 L49 makes body 26 at (3.6273, 11.1689, 1.4667) makes body 27 at (-8.4995, 10.5822, 1.4667) makes body 28 at (13.5356, 9.6319, 1.4667) makes body 29 at (-0.5171, 11.2107, 1.4667) makes body 30 at (-4.4409, 10.5822, 1.4667) makes body 31 at (15.029, 9.6815, 1.4667)
extrude "Extrude5" add sketch "Sketch1" along normal blind 2.1 separate body contours A6 | A7 | A8 makes body 32 at (9.3641, 9.7877, 0.7) makes body 33 at (-11.322, 9.2789, 0.7) makes body 34 at (-15.3825, 9.2907, 0.7)
extrude "Extrude6" add sketch "Sketch1" along normal blind 8 separate body contours A0 makes body 35
extrude "Extrude7" add sketch "Sketch1" along normal blind 7.5 separate body contours A1 makes body 36
extrude "Extrude8" add sketch "Sketch1" along normal blind 7 separate body contours L50 L51 L52 L53 makes body 37
extrude "Extrude9" add sketch "Sketch1" along normal blind 5 separate body contours L22 L24 A2 A3 A4 A5 makes body 38
extrude "Extrude10" add sketch "Sketch1" along normal blind 10 separate body contours L10 L11 L12 L13 makes body 39
extrude "Extrude11" add sketch "Sketch1" along normal blind 6 separate body contours L6 L7 L8 L9 L19 L20 L21 makes body 40
extrude "Extrude12" add sketch "Sketch1" along normal blind 3 separate body contours L8 L18 L19 L21 | L14 L15 L16 L17 makes body 41 at (-5.3822, -3.1736, 1) makes body 42 at (12.1467, -9.3154, 1)

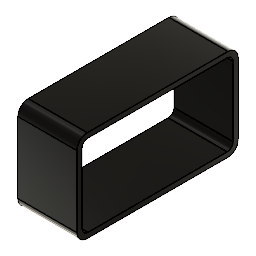
design "Battery Strap"
Autodesk Fusion 360 part; units mm, degrees
sketch "Sketch1" plane through (0, 0, 0) normal (1, 0, 0) x (0, 1, 0)
  line L0 (23.5, -13.75) -> (-23.5, -13.75)
  line L1 (-25.5, -11.75) -> (-25.5, 11.75)
  line L2 (-23.5, 13.75) -> (23.5, 13.75)
  line L3 (25.5, 11.75) -> (25.5, -11.75)
  line L4 (25.5, -13.75) -> (-25.5, 13.75) construction
  line L5 (-25.5, -13.75) -> (25.5, 13.75) construction
  line L6 (23.75, -15.5) -> (-23.75, -15.5)
  line L7 (-27.25, -12) -> (-27.25, 12)
  line L8 (-23.75, 15.5) -> (23.75, 15.5)
  line L9 (27.25, 12) -> (27.25, -12)
  line L10 (27.25, -15.5) -> (-27.25, 15.5) construction
  line L11 (-27.25, -15.5) -> (27.25, 15.5) construction
  arc A0 (27.25, 12) -> (23.75, 15.5) centre (23.75, 12) ccw
  arc A1 (23.75, -15.5) -> (27.25, -12) centre (23.75, -12) ccw
  arc A2 (-27.25, -12) -> (-23.75, -15.5) centre (-23.75, -12) ccw
  arc A3 (-23.75, 15.5) -> (-27.25, 12) centre (-23.75, 12) ccw
  arc A4 (-23.5, 13.75) -> (-25.5, 11.75) centre (-23.5, 11.75) ccw
  arc A5 (25.5, 11.75) -> (23.5, 13.75) centre (23.5, 11.75) ccw
  arc A6 (23.5, -13.75) -> (25.5, -11.75) centre (23.5, -11.75) ccw
  arc A7 (-25.5, -11.75) -> (-23.5, -13.75) centre (-23.5, -11.75) ccw
  dimension "d1" = 51
  dimension "d2" = 27.5
  dimension "d3" = 54.5
  dimension "d4" = 31
  dimension "d7" = 3.5
  dimension "d8" = 3.5
  dimension "d9" = 3.5
  dimension "d10" = 3.5
  dimension "d11" = 2
  dimension "d12" = 2
  dimension "d13" = 2
  dimension "d14" = 2
  measures "d7" radius of A0
  measures "d8" radius of A1
  measures "d9" radius of A2
  measures "d10" radius of A3
  measures "d11" radius of A4
  measures "d12" radius of A5
  measures "d13" radius of A6
  measures "d14" radius of A7
extrude "Extrude1" add sketch "Sketch1" along normal mid plane 20
equation "d3 = 51 mm + 1.75 mm + 1.75 mm"
equation "d4 = 27.5 mm + 1.75 mm + 1.75 mm"
named bodies: "Battery Strap"

design "624Z Bearing"
Autodesk Fusion 360 part; units mm, degrees
sketch "Sketch1" plane through (0.0608, -5, -3.3084) normal (0, -1, 0) x (1, 0, 0)
  circle A0 centre (9.4392, 13.5084) radius 6.5
  circle A1 centre (9.4392, 13.5084) radius 2
  circle A2 centre (9.4392, 13.5084) radius 3
  circle A3 centre (9.4392, 13.5084) radius 5.5
  circle A4 centre (9.4392, 13.5084) radius 5.2
  circle A5 centre (9.4392, 13.5084) radius 3.25
  dimension "d44" = 13
  dimension "d45" = 4
  dimension "d46" = 6
  dimension "d47" = 11
  dimension "d48" = 10.4
  dimension "d49" = 6.5
  dimension "d56" = 0
  dimension "d57" = 0
  dimension "d58" = 0
  dimension "d59" = 0
  dimension "d68" = 0
  dimension "d69" = 0
  dimension "d70" = 0
  dimension "d71" = 0
  measures "d44" diameter of A0
  measures "d45" diameter of A1
  measures "d46" diameter of A2
  measures "d47" diameter of A3
  measures "d48" diameter of A4
  measures "d49" diameter of A5
extrude "Extrude1" add sketch "Sketch1" along normal mid plane 5 contours A0 | A2 makes body 1 at (15.9919, -6.6667, 9.876) makes body 2 at (12.4963, -6.6667, 10.0505)
extrude "Extrude2" add sketch "Sketch1" along normal mid plane 4.8 separate body contours A4 makes body 3
extrude "Extrude3" add sketch "Sketch1" along normal mid plane 4.6 contours A3 | A5 bodies 1 2 3
chamfer "Chamfer1" distance 0.1 angle 45 4 edges at (3.4399, -7.5, 7.8495) (3.4399, -2.5, 12.5505) (7.6353, -7.5, 10.9232) (7.6353, -2.5, 9.4768) on bodies 1
